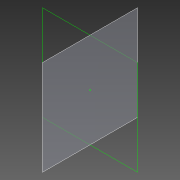
# Autodesk Inventor part: Sentroller_Mount
Saved by Autodesk Inventor 2017 (Build 210142000, 142)
## iProperties
Created: 2016-08-31
Part Number: Sentroller_Mount
Material: Generic
Document SubType Name: Modeling
Designer: Dmitry
Density: 1 g/cm^3
Appearance: Default
Author: Dmitry
Autodesk Inventor part; units mm, degrees
ref_plane "YZ Plane" through (0, 0, 0) normal (1, 0, 0) x (0, 1, 0)
ref_plane "XZ Plane" through (0, 0, 0) normal (0, 1, 0) x (-1, 0, 0)
ref_plane "XY Plane" through (0, 0, 0) normal (0, 0, 1) x (1, 0, 0)
ref_plane "Work Plane2" through (0, 0, 0) normal (1, 0, 0) x (0, 0, -1)
sketch "Sketch1" plane through (0, 0, 0) normal (1, 0, 0) x (0, 0, -1)
  line L0 (20, -35) -> (-20, -35)
  line L1 (-20, -35) -> (-20, 35)
  line L2 (-20, 35) -> (20, 35)
  line L3 (20, 35) -> (20, -35)
  line L4 (20, -35) -> (-20, 35) construction
  line L5 (-20, -35) -> (20, 35) construction
  point P0 (0, 0)
  dimension "d0" = 40
  dimension "d1" = 70
  constraints: 12 end point, 2 midpoint, 2 parallel, 1 horizontal, 1 perpendicular
  measures "d0" distance of L1.end L2.end
  measures "d1" distance of L0.end L1.end
extrude "Extrusion1" add sketch "Sketch1" along normal blind 5
fillet "Fillet1" radius 12.25 4 edges at (2.5, -35, 20) (2.5, -35, -20) (2.5, 35, -20) (2.5, 35, 20)
sketch "Sketch2" plane through (0, 0, 0) normal (-1, 0, 0) x (0, 0, 1)
  circle A0 centre (0, -16.7815) radius 6.6
  line L0 (30.2912, 0) -> (32.4021, 0)
  circle A1 centre (0, 16.7815) radius 6.6
  point P0 (0, 0)
  dimension "d5" = 13.2
  constraints: 2 centre point, 2 end point, 1 horizontal, 1 symmetric about line, 1 other
  measures "d5" diameter of A0
extrude "Extrusion2" cut sketch "Sketch2" against normal blind 3.75
sketch "Sketch3" plane through (0, 0, 0) normal (-1, 0, 0) x (0, 0, 1)
  circle A0 centre (0, 16.7815) radius 6.6 projected
  circle A1 centre (0, -16.7815) radius 6.6 projected
  point P0 (0, 0)
extrude "Extrusion3" add sketch "Sketch3" against normal blind 0.4
sketch "Sketch4" plane through (5, 0, 0) normal (1, 0, 0) x (0, 0, -1)
  line L0 (13, -26.7517) -> (-13, -26.7517)
  line L1 (-13, -26.7517) -> (-13, 18.2483)
  line L2 (-13, 18.2483) -> (13, 18.2483)
  line L3 (13, 18.2483) -> (13, -26.7517)
  line L4 (13, -26.7517) -> (-13, 18.2483) construction
  line L5 (-13, -26.7517) -> (13, 18.2483) construction
  point P0 (0, -4.2517)
  point P1 (0, 0)
  dimension "d10" = 26
  dimension "d11" = 45
  dimension "d12" = 0
  constraints: 12 end point, 2 midpoint, 2 parallel, 1 horizontal, 1 perpendicular, 1 other
  measures "d10" distance of L1.end L2.end
  measures "d11" distance of L0.end L1.end
  measures "d12" horizontal distance of point (0, 0) point (0, -4.252)
extrude "Extrusion4" cut sketch "Sketch4" against normal blind 0.4
body "Solid1"
